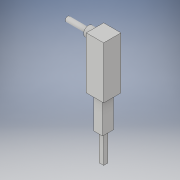
# Autodesk Inventor part: simp_burnisher
Saved by Autodesk Inventor 2019 (Build 230136000, 136)
## iProperties
Created: 2019-11-07
Part Number: simp_burnisher
Material: Generic
Document SubType Name: Modeling
Designer: luua
Density: 1 g/cm^3
Appearance: Default
Author: luua
Autodesk Inventor part; units mm, degrees
ref_plane "YZ Plane" through (0, 0, 0) normal (1, 0, 0) x (0, 1, 0)
ref_plane "XZ Plane" through (0, 0, 0) normal (0, 1, 0) x (-1, 0, 0)
ref_plane "XY Plane" through (0, 0, 0) normal (0, 0, 1) x (1, 0, 0)
sketch "Sketch1" plane through (0, 0, 0) normal (0, 0, 1) x (1, 0, 0)
  line L0 (-76.6085, 0) -> (76.6085, 0) construction
  line L1 (-48, 0) -> (48, 0)
  line L2 (48, 0) -> (48, 11)
  line L3 (48, 11) -> (-48, 11)
  line L4 (-48, 11) -> (-48, 0)
  point P0 (0, 0)
  point P1 (0, 0)
  point P2 (0, 11)
  dimension "d0" = 96
  dimension "d1" = 11
  constraints: 10 end point, 2 horizontal, 2 midpoint, 2 parallel, 1 coincident, 1 perpendicular, 1 point on line, 1 vertical alignment
  measures "d0" distance of L2.end L3.end
  measures "d1" distance of L1.end L2.end
revolve "Revolution1" add sketch "Sketch1" angle 360 about axis through (-76.6085, 0, 0) along (1, 0, 0)
sketch "Sketch2" plane through (48, 0, 0) normal (1, 0, 0) x (0, 0, -1)
  circle A0 centre (0, 0) radius 22.5
  dimension "d3" = 45
  constraints: 1 centre point, 1 coincident
  measures "d3" diameter of A0
extrude "Extrusion1" add sketch "Sketch2" along normal blind 30
sketch "Sketch3" plane through (0, 0, 0) normal (0, 0, 1) x (1, 0, 0)
  line L0 (78, -22.5) -> (78, 22.5) projected
  line L1 (78, 27.5) -> (78, -212.5)
  line L2 (48, 22.5) -> (78, 22.5) projected
  line L3 (48, -22.5) -> (78, -22.5) projected
  line L4 (78, 27.5) -> (158, 27.5)
  line L5 (158, 27.5) -> (158, -212.5)
  line L6 (78, -212.5) -> (98, -212.5)
  line L7 (158, -212.5) -> (138, -212.5)
  line L8 (118, 27.5) -> (118, -212.5) construction
  line L9 (98, -212.5) -> (98, -362.5)
  line L10 (98, -362.5) -> (138, -362.5)
  line L11 (138, -362.5) -> (138, -212.5)
  line L12 (108, -362.5) -> (128, -362.5)
  line L13 (128, -362.5) -> (128, -492.5)
  line L14 (128, -492.5) -> (108, -492.5)
  line L15 (108, -492.5) -> (108, -362.5)
  line L16 (138, -212.5) -> (98, -212.5)
  point P0 (0, 0)
  point P1 (118, -362.5)
  dimension "d6" = 5
  dimension "d7" = 190
  dimension "d8" = 80
  dimension "d9" = 40
  dimension "d10" = 150
  dimension "d36" = 20
  dimension "d37" = 130
  constraints: 28 end point, 6 horizontal, 3 midpoint, 3 perpendicular, 3 vertical, 2 collinear, 2 parallel, 1 horizontal alignment, 1 symmetric about line
  measures "d6" distance from line of L1.start L2
  measures "d7" distance from line of L1.end L3
  measures "d8" distance of L1.start L4.end
  measures "d9" distance of L6.end L7.end
  measures "d10" distance of L6.end L9.end
  measures "d36" distance of L13.end L14.end
  measures "d37" distance of L12.end L13.end
extrude "Extrusion2" add sketch "Sketch3" along normal mid plane 80 contours L0 L1 L4 L5 L7 L16 L6
extrude "Extrusion7" add sketch "Sketch3" along normal mid plane 50 contours L16 L11 L10 L9
extrude "Extrusion8" add sketch "Sketch3" along normal mid plane 20 contours L10 L13 L14 L15
body "Solid1"
